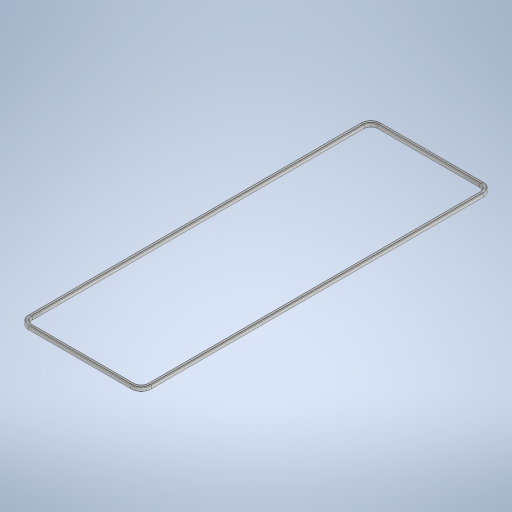
# Autodesk Inventor part: LI0005-SEAL
Saved by Autodesk Inventor 2023 (Build 270158000, 158)
## iProperties
Created: 2023-03-15
Part Number: LI0005-SEAL
Material: Generic
Document SubType Name: Modeling
Designer: Louis
Density: 1 g/cm^3
Appearance: Default
Author: Louis
Autodesk Inventor part; units mm, degrees
ref_plane "YZ Plane" through (0, 0, 0) normal (1, 0, 0) x (0, 1, 0)
ref_plane "XZ Plane" through (0, 0, 0) normal (0, 1, 0) x (-1, 0, 0)
ref_plane "XY Plane" through (0, 0, 0) normal (0, 0, 1) x (1, 0, 0)
sketch "Sketch1" plane through (0, 0, 0) normal (0, 1, 0) x (-1, 0, 0)
  circle A0 centre (60, 195) radius 12
  circle A1 centre (60, -195) radius 12
  circle A2 centre (-60, 195) radius 12
  circle A3 centre (-60, -195) radius 12
  line L0 (72, 195) -> (72, -195)
  line L1 (60, -207) -> (-60, -207)
  line L2 (60, 207) -> (-60, 207)
  line L3 (-72, 195) -> (-72, -195)
  line L4 (68, 195) -> (68, -195)
  circle A4 centre (60, 195) radius 8
  line L5 (60, 203) -> (-60, 203)
  circle A5 centre (-60, 195) radius 8
  line L6 (-68, 195) -> (-68, -195)
  circle A6 centre (-60, -195) radius 8
  line L7 (60, -203) -> (-60, -203)
  circle A7 centre (60, -195) radius 8
  point P0 (0, 0)
  point P1 (72, 0)
  point P2 (0, 207)
  point P3 (35, 143)
  point P4 (68, 135)
  point P5 (68, -135)
  point P6 (35, -143)
  point P7 (-60, -203)
  point P8 (-68, -135)
  point P9 (-68, 135)
  point P10 (-60, 203)
  dimension "d0" = 24
  dimension "d1" = 24
  dimension "d2" = 24
  dimension "d3" = 24
  dimension "d6" = 4
  dimension "d7" = 4
  dimension "d8" = 4
  dimension "d9" = 4
  dimension "d10" = 4
  dimension "d11" = 4
  dimension "d12" = 4
  dimension "d13" = 4
  dimension "d35" = 414
  dimension "d36" = 144
  constraints: 16 end point, 12 point on circle, 6 centre point, 6 parallel, 6 tangent, 3 horizontal alignment, 3 vertical alignment, 2 midpoint, 6 other
  measures "d0" diameter of A0
  measures "d1" diameter of A2
  measures "d2" diameter of A1
  measures "d3" diameter of A3
  measures "d6" distance between parallel lines of L0 L4
  measures "d7" radial gap between concentric circles of A0 A4
  measures "d8" distance between parallel lines of L2 L5
  measures "d10" distance between parallel lines of L3 L6
  measures "d12" distance between parallel lines of L1 L7
  measures "d13" radial gap between concentric circles of A1 A7
  measures "d35" distance between parallel lines of L1 L2
  measures "d36" distance between parallel lines of L3 L0
extrude "Extrusion1" add sketch "Sketch1" along normal blind 4.5 contours A0 L4 A4 L5 | L0 A1 L4 A0 | A0 L5 A2 L2 | A1 L7 A7 L4 | A2 L5 A5 L6 | L1 A3 L7 A1 | A2 L6 A3 L3 | A3 L6 A6 L7 picked at (54.6594, 203.5636) picked at (54.6594, -203.5636) picked at (-54.6594, 203.5636) picked at (-54.6594, -203.5636)
sketch "Sketch2" plane through (0, 4.5, 0) normal (0, 1, 0) x (1, 0, 0)
  line L0 (-72, 195) -> (-72, -195) projected
  arc A0 (-72, -195) -> (-60, -207) centre (-60, -195) ccw projected
  line L1 (-60, -207) -> (60, -207) projected
  arc A1 (60, -207) -> (72, -195) centre (60, -195) ccw projected
  line L2 (72, -195) -> (72, 195) projected
  arc A2 (72, 195) -> (60, 207) centre (60, 195) ccw projected
  line L3 (60, 207) -> (-60, 207) projected
  arc A3 (-60, 207) -> (-72, 195) centre (-60, 195) ccw projected
  line L4 (-69.5, -195) -> (-69.5, 195)
  arc A4 (-60, 204.5) -> (-69.5, 195) centre (-60, 195) ccw
  line L5 (-60, 204.5) -> (60, 204.5)
  arc A5 (69.5, 195) -> (60, 204.5) centre (60, 195) ccw
  line L6 (69.5, 195) -> (69.5, -195)
  arc A6 (60, -204.5) -> (69.5, -195) centre (60, -195) ccw
  line L7 (60, -204.5) -> (-60, -204.5)
  arc A7 (-69.5, -195) -> (-60, -204.5) centre (-60, -195) ccw
  line L8 (-70.5, -195) -> (-70.5, 195)
  arc A8 (-60, 205.5) -> (-70.5, 195) centre (-60, 195) ccw
  line L9 (-60, 205.5) -> (60, 205.5)
  arc A9 (70.5, 195) -> (60, 205.5) centre (60, 195) ccw
  line L10 (70.5, 195) -> (70.5, -195)
  arc A10 (60, -205.5) -> (70.5, -195) centre (60, -195) ccw
  line L11 (60, -205.5) -> (-60, -205.5)
  arc A11 (-70.5, -195) -> (-60, -205.5) centre (-60, -195) ccw
  point P0 (0, 0)
  dimension "d16" = 2.5
  dimension "d17" = 1.5
  constraints: 16 end point, 16 point on circle, 8 centre point, 14 other
  measures "d16" distance between parallel lines of L0 L4
  measures "d17" distance between parallel lines of L0 L8
extrude "Extrusion2" cut sketch "Sketch2" against normal blind 1 contours L8 A8 L9 A9 L10 A10 L11 A11
chamfer "Chamfer3" distance 0.5 distance2 1 8 edges at (0, 4.5, 205.5) (-67.4246, 4.5, 202.4246) (-70.5, 4.5, 0) (-67.4246, 4.5, -202.4246) (0, 4.5, -205.5) (67.4246, 4.5, -202.4246) (70.5, 4.5, 0) (67.4246, 4.5, 202.4246) measured on face at (-71, 4.5, 65)
chamfer "Chamfer4" distance 0.5 distance2 1 8 edges at (0, 4.5, 204.5) (66.7175, 4.5, 201.7175) (69.5, 4.5, 0) (66.7175, 4.5, -201.7175) (0, 4.5, -204.5) (-66.7175, 4.5, -201.7175) (-69.5, 4.5, 0) (-66.7175, 4.5, 201.7175) measured on face at (-69, 4.5, -65)
chamfer "Chamfer5" distance 0.5 angle 45 32 edges at (0, 4.5, 207) (68.4853, 4.5, 203.4853) (72, 4.5, 0) (68.4853, 4.5, -203.4853) (0, 4.5, -207) (-68.4853, 4.5, -203.4853) (-72, 4.5, 0) (-68.4853, 4.5, 203.4853) (0, 4.5, 203) (-65.6569, 4.5, 200.6569) (-68, 4.5, 0) (-65.6569, 4.5, -200.6569) (0, 4.5, -203) (65.6569, 4.5, -200.6569) (68, 4.5, 0) (65.6569, 4.5, 200.6569) (68.4853, 0, 203.4853) (72, 0, 0) (68.4853, 0, -203.4853) (0, 0, -207) (-68.4853, 0, -203.4853) (-72, 0, 0) (-68.4853, 0, 203.4853) (0, 0, 207) (0, 0, 203) (-65.6569, 0, 200.6569) (-68, 0, 0) (-65.6569, 0, -200.6569) (0, 0, -203) (65.6569, 0, -200.6569) (68, 0, 0) (65.6569, 0, 200.6569)
body "Solid1"
